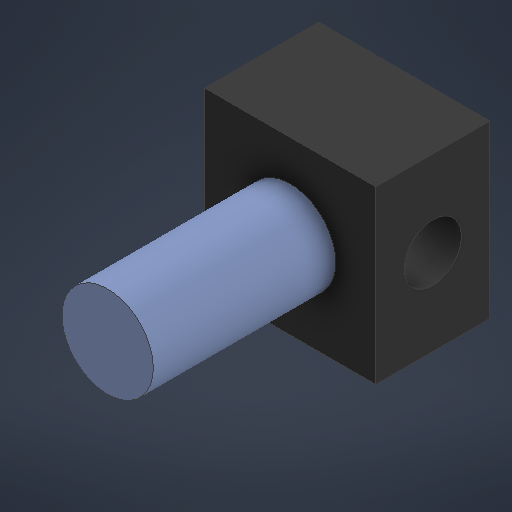
# Autodesk Inventor part: Diastal
Saved by Autodesk Inventor 2026 (Build 300175000, 175)
## iProperties
Created: 2026-01-04
Part Number: Diastal
Material: Generic
Document SubType Name: Modeling
Designer: saraswat22
Density: 1 g/cm^3
Appearance: Default
Author: saraswat22
Autodesk Inventor part; units mm, degrees
ref_plane "YZ Plane" through (0, 0, 0) normal (1, 0, 0) x (0, 1, 0)
ref_plane "XZ Plane" through (0, 0, 0) normal (0, 1, 0) x (-1, 0, 0)
ref_plane "XY Plane" through (0, 0, 0) normal (0, 0, 1) x (1, 0, 0)
sketch "Sketch1" plane through (0, 0, 0) normal (0, 0, 1) x (1, 0, 0)
  line L0 (-76.2, -76.2) -> (76.2, -76.2)
  line L1 (76.2, -76.2) -> (76.2, 76.2)
  line L2 (76.2, 76.2) -> (-76.2, 76.2)
  line L3 (-76.2, 76.2) -> (-76.2, -76.2)
  line L4 (-76.2, -76.2) -> (76.2, 76.2) construction
  line L5 (76.2, -76.2) -> (-76.2, 76.2) construction
  point P0 (0, 0)
  dimension "d0" = 152.4
  dimension "d1" = 152.4
  constraints: 12 end point, 2 midpoint, 2 parallel, 1 horizontal, 1 perpendicular
  measures "d0" distance of L2.end L1.end
  measures "d1" distance of L1.end L0.end
extrude "Extrusion1" add sketch "Sketch1" along normal blind 101.6
sketch "Sketch2" plane through (0, 0, 101.6) normal (0, 0, 1) x (1, 0, 0)
  circle A0 centre (0, 0) radius 40.64
  dimension "d4" = 81.28
  constraints: 1 centre point, 1 coincident
  measures "d4" diameter of A0
extrude "Extrusion2" add sketch "Sketch2" along normal blind 162.56
sketch "Sketch3" plane through (76.2, -76.2, 0) normal (1, 0, 0) x (0, 0, -1)
  circle A0 centre (-50.8, 76.2) radius 25.4
  point P0 (0, 76.2)
  dimension "d7" = 50.8
  constraints: 1 centre point
  measures "d7" diameter of A0
extrude "Extrusion3" cut sketch "Sketch3" against normal through all
body "Solid1"
